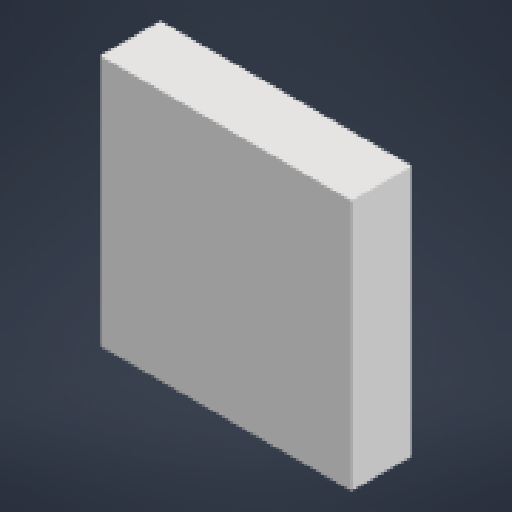
# Autodesk Inventor part: light box
Saved by Autodesk Inventor 2024 (Build 280153000, 153)
## iProperties
Created: 2023-07-17
Part Number: light box
Material: 일반
Document SubType Name: Modeling
Designer: wodyd
Mass: 4.42 g
Surface Area: 71.2 cm^2
Volume: 4.42 cm^3
Density: 1 g/cm^3
Appearance: 기본값
Author: wodyd
Autodesk Inventor part; units mm, degrees
ref_plane "YZ Plane" through (0, 0, 0) normal (1, 0, 0) x (0, 1, 0)
ref_plane "XZ Plane" through (0, 0, 0) normal (0, 1, 0) x (-1, 0, 0)
ref_plane "XY Plane" through (0, 0, 0) normal (0, 0, 1) x (1, 0, 0)
sketch "스케치1" plane through (0, 0, 0) normal (0, 0, 1) x (1, 0, 0)
  line L0 (25, 25) -> (-25, 25) projected
  line L1 (-25, 25) -> (-25, -25) projected
  line L2 (-25, -25) -> (25, -25) projected
  line L3 (25, -25) -> (25, 25) projected
  line L4 (-23, 23) -> (23, 23)
  line L5 (23, 23) -> (23, -23)
  line L6 (23, -23) -> (-23, -23)
  line L7 (-23, -23) -> (-23, 23)
  point P0 (0, 0)
  dimension "d0" = 2
  constraints: 8 end point, 3 other
  measures "d0" distance between parallel lines of L0 L4
extrude "돌출1" add sketch "스케치1" along normal blind 5
sketch "스케치2" plane through (0, 0, 5) normal (0, 0, 1) x (1, 0, 0)
  line L0 (25, 25) -> (-25, 25) projected
  line L1 (-25, 25) -> (-25, -25) projected
  line L2 (-25, -25) -> (25, -25) projected
  line L3 (25, -25) -> (25, 25) projected
  point P0 (0, 0)
extrude "돌출2" add sketch "스케치2" along normal blind 1
